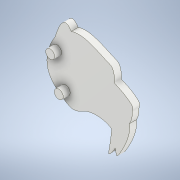
# Autodesk Inventor part: Component18
Saved by Autodesk Inventor 2022 (Build 260153000, 153)
## iProperties
Created: 2022-01-29
Part Number: Component18
Material: Generic
Document SubType Name: Modeling
Designer: Administrator
Density: 1 g/cm^3
Appearance: Default
Title: Component18
Author: Administrator
Autodesk Inventor part; units mm, degrees
ref_plane "YZ Plane" through (0, 0, 0) normal (1, 0, 0) x (0, 1, 0)
ref_plane "XZ Plane" through (0, 0, 0) normal (0, 1, 0) x (-1, 0, 0)
ref_plane "XY Plane" through (0, 0, 0) normal (0, 0, 1) x (1, 0, 0)
sketch "Sketch2" plane through (0, 0, 0) normal (0, 0, 1) x (1, 0, 0)
  circle A0 centre (-29.626, -25.6418) radius 3.25
  circle A1 centre (-35.8614, -3.5337) radius 3.25
  spline S0 degree 5 poles (-37.3245, 3.9247) (-37.9121, 3.0606) (-39.234, 0.9409) (-41.0264, -2.6059) (-42.7739, -7.6359) (-43.6073, -13.7371) (-42.7953, -19.355) (-40.0321, -24.3495) (-35.7762, -28.7263) (-30.9799, -32.228) (-27.5735, -34.0731) (-25.6696, -34.7855) (-24.7441, -34.9438) (-24.3673, -34.9438) knots -0.290868 -0.290868 -0.290868 -0.290868 -0.290868 -0.290868 -0.266667 -0.233333 -0.2 -0.166667 -0.133333 -0.1 -0.066667 -0.033333 0 0 0 0 0 0 weights 1 1 1 1 1 1 1 1 1 1 1 1 1 1
  spline S1 degree 5 poles (-24.3673, -34.9438) (-23.6544, -34.9438) (-22.3157, -34.8458) (-20.5687, -34.4047) (-18.6026, -33.331) (-15.9544, -31.7223) (-12.4416, -30.4472) (-7.7506, -29.9919) (-2.8402, -30.4321) (0.1572, -31.2555) (1.8356, -32.0636) (2.8609, -32.6759) (3.4348, -33.0364) (3.5797, -33.1282) knots 0 0 0 0 0 0 0.1 0.2 0.3 0.4 0.5 0.6 0.7 0.8 0.833862 0.833862 0.833862 0.833862 0.833862 0.833862 weights 1 1 1 1 1 1 1 1 1 1 1 1 1 1
  spline S2 degree 5 poles (3.5797, -33.1282) (3.5829, -33.784) (3.557, -35.1326) (3.4213, -37.2661) (3.067, -40.2732) (2.4677, -43.9587) (1.8929, -47.1321) (1.5592, -49.3501) (1.6664, -50.2794) (2.4345, -49.7586) (3.942, -47.9825) (5.4445, -45.7682) (6.2931, -44.0978) (6.2623, -43.8572) (6.586, -45.5178) (7.1881, -47.7238) (7.59, -48.6899) (8.1689, -48.0278) (9.3852, -46.0931) (11.137, -43.0269) (13.1742, -39.1316) (15.0908, -34.7167) (16.4105, -30.3901) (16.8796, -27.1883) (16.8756, -25.1213) (16.7581, -23.9739) (16.6888, -23.517) knots 0 0 0 0 0 0 0.04 0.08 0.12 0.16 0.2 0.24 0.28 0.32 0.36 0.4 0.44 0.48 0.52 0.56 0.6 0.64 0.68 0.72 0.76 0.8 0.84 0.869987 0.869987 0.869987 0.869987 0.869987 0.869987 weights 1 1 1 1 1 1 1 1 1 1 1 1 1 1 1 1 1 1 1 1 1 1 1 1 1 1 1
  spline S3 degree 5 poles (16.6888, -23.517) (17.1279, -22.6782) (18.0311, -20.7168) (18.7115, -18.2364) (18.5946, -16.0826) (18.3426, -14.7145) (19.2913, -13.6847) (19.6674, -11.7304) (15.2871, -8.1346) (9.3469, -4.8731) (5.3779, -3.3884) (5.9012, -3.7581) (6.1075, -0.5295) (5.0558, 4.3106) (3.5561, 6.4103) (1.3258, 7.0143) (-2.2903, 8.5843) (-7.1686, 10.898) (-13.0363, 13.3353) (-18.1182, 14.4122) (-21.9097, 14.2882) (-24.3686, 13.7542) (-25.5749, 13.3747) (-25.5768, 13.3741) knots -0.954926 -0.954926 -0.954926 -0.954926 -0.954926 -0.954926 -0.933333 -0.9 -0.866667 -0.833333 -0.8 -0.766667 -0.733333 -0.7 -0.666667 -0.633333 -0.6 -0.566667 -0.533333 -0.5 -0.466667 -0.433333 -0.4 -0.366667 -0.366616 -0.366616 -0.366616 -0.366616 -0.366616 -0.366616 weights 1 1 1 1 1 1 1 1 1 1 1 1 1 1 1 1 1 1 1 1 1 1 1 1
  spline S4 degree 5 poles (-25.5768, 13.3741) (-25.6989, 13.5664) (-26.0858, 14.1555) (-26.7345, 15.0372) (-27.6396, 16.0101) (-28.7924, 16.7562) (-30.0653, 16.8917) (-31.3182, 16.2988) (-32.5519, 15.0053) (-33.7681, 13.0728) (-34.9685, 10.5673) (-35.9175, 8.1495) (-36.6232, 6.1199) (-37.0912, 4.6722) (-37.3245, 3.9247) knots 0.053969 0.053969 0.053969 0.053969 0.053969 0.053969 0.1 0.2 0.3 0.4 0.5 0.6 0.7 0.8 0.9 1 1 1 1 1 1 weights 1 1 1 1 1 1 1 1 1 1 1 1 1 1 1
  point P0 (0, 0)
  point P1 (30.6979, -34.6022)
  dimension "d4" = 6.5
  constraints: 2 centre point, 1 equal radius, 10 other
  measures "d4" diameter of A1
extrude "Extrusion1" add sketch "Sketch2" against normal blind 5 contours A0 | A1 | S4 S3 S2 S1 S0
extrude "Extrusion2" add sketch "Sketch2" along normal blind 5 contours A0 | A1
equation "\"d4\" = R"
equation "\"R\" = 6.5"
equation "\"thickness\" = 5"
equation "\"width\" = 6.5"
equation "\"R1\" = 9"
body "Solid1"
